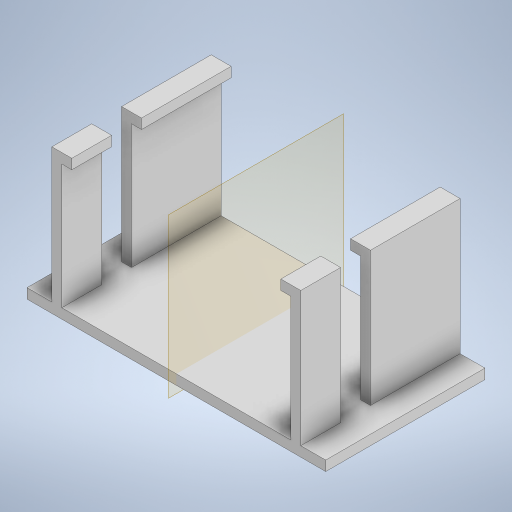
# Autodesk Inventor part: ServoHalterung
Saved by Autodesk Inventor 2023.1 (Build 271208000, 208)
## iProperties
Created: 2023-04-24
Part Number: ServoHalterung
Material: Generisch
Document SubType Name: Sheet Metal
Designer: marco
Density: 1 g/cm^3
Sheet Metal Rule: Standard_mm
Appearance: Vorgabe
Author: marco
Autodesk Inventor part; units mm, degrees
ref_plane "YZ Plane" through (0, 0, 0) normal (1, 0, 0) x (0, 1, 0)
ref_plane "XZ Plane" through (0, 0, 0) normal (0, 1, 0) x (-1, 0, 0)
ref_plane "XY Plane" through (0, 0, 0) normal (0, 0, 1) x (1, 0, 0)
sketch "Skizze1" plane through (0, 0, 0) normal (0, 1, 0) x (-1, 0, 0)
  line L0 (0, 0) -> (30, 0)
  line L1 (30, 0) -> (30, -16)
  line L2 (30, -16) -> (0, -16)
  line L3 (0, -16) -> (0, 0)
  dimension "d0" = 30
  dimension "d1" = 16
  constraints: 8 end point, 2 parallel, 1 horizontal, 1 perpendicular
  measures "d0" distance of L1.end L2.end
  measures "d1" distance of L0.end L1.end
extrude "Extrusion1" add sketch "Skizze1" along normal blind 1
sketch "Skizze2" plane through (-30, 0, 0) normal (0, 0, 1) x (1, 0, 0)
  line L0 (30, 1) -> (0, 1) projected
  line L1 (27.5, 1) -> (27.5, 14.5)
  line L2 (27.5, 1) -> (41, 1) construction
  line L3 (27.5, 14.5) -> (25.5, 14.5)
  line L4 (25.5, 14.5) -> (25.5, 13.5)
  line L5 (25.5, 13.5) -> (26.5, 13.5)
  line L6 (26.5, 13.5) -> (26.5, 1)
  line L7 (26.5, 1) -> (27.5, 1)
  line L8 (15, 1) -> (15, 5.7863)
  point P0 (30, 0)
  point P1 (15, 3.3931)
  point P2 (26.5, 1)
  dimension "d4" = 13.5
  dimension "d5" = 90
  dimension "d6" = 2
  dimension "d7" = 1
  dimension "d8" = 1
  dimension "d9" = 11.5
  constraints: 16 end point, 7 perpendicular, 2 midpoint, 1 horizontal, 1 point on line, 1 vertical
  measures "d4" distance of L1.start L1.end
  measures "d5" angle of L2 L1
  measures "d6" distance of L1.end L3.end
  measures "d7" distance of L3.end L4.end
  measures "d8" distance of L4.end L5.end
  measures "d9" distance from line of point (15, 3.393) L6
extrude "Extrusion2" add sketch "Skizze2" against normal blind 16
ref_plane "Arbeitsebene1" through (-15, 0, 0) normal (1, 0, 0) x (0, 0, -1)
sketch "Skizze3" plane through (-2.5, 1, 0) normal (1, 0, 0) x (0, 0, -1)
  line L0 (16, 0) -> (0, 0) projected
  line L1 (4, 0) -> (7, 0)
  line L2 (7, 0) -> (7, 14.6067)
  line L3 (7, 14.6067) -> (4, 14.6067)
  line L4 (4, 14.6067) -> (4, 0)
  point P0 (0, -1)
  point P1 (7, 0)
  dimension "d12" = 3
  constraints: 8 end point, 2 parallel, 1 horizontal, 1 perpendicular, 1 point on line
  measures "d12" distance of L3.end L2.end
extrude "Extrusion3" cut sketch "Skizze3" against normal blind 16
mirror "Spiegeln1" about plane through (-15, 0, 0) normal (1, 0, 0) of "Extrusion2", "Extrusion3"
equation "\"Biegeradius\" = Stärke"
equation "\"BreiteBiegungsfreistellung\" = Stärke"
equation "\"TiefeBiegungsfreistellung\" = 0.5 * Stärke"
equation "\"GrößeEckenfreistellung\" = 4 * Stärke"
equation "\"MinimalRest\" = 2 * Stärke"
equation "\"Übergangsradius\" = Biegeradius"
equation "\"JacobiRadiusGröße\" = Biegeradius"
equation "\"Abstandsgröße\" = Stärke"
equation "\"Stärke\" = 0.5"
